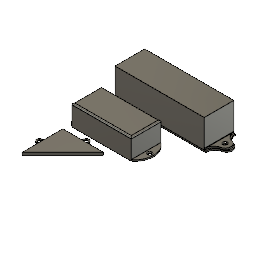
Glow_casings v2 (Autodesk Fusion 360 design; units mm, degrees)
Autodesk Fusion 360 part; units mm, degrees
sketch "Electronic case cap - sketch" plane through (0, 0, 0) normal (0, 1, 0) x (1, 0, 0)
  line L0 (0, 0) -> (137, 0)
  line L1 (0, 0) -> (0, -137)
  line L2 (0, -137) -> (137, 0)
  line L3 (68.5, 0) -> (58.5, 0)
  line L4 (58.5, 0) -> (58.5, 20)
  line L5 (58.5, 20) -> (68.5, 20)
  line L6 (68.5, 20) -> (68.5, 0)
  line L7 (68.5, 0) -> (78.5, 0)
  line L8 (78.5, 0) -> (78.5, 20)
  line L9 (78.5, 20) -> (68.5, 20)
  line L10 (68.5, 20) -> (68.5, 0)
  line L11 (0, -68.5) -> (-20, -68.5)
  line L12 (-20, -68.5) -> (-20, -78.5)
  line L13 (-20, -78.5) -> (0, -78.5)
  line L14 (0, -78.5) -> (0, -68.5)
  line L15 (0, -68.5) -> (-20, -68.5)
  line L16 (-20, -68.5) -> (-20, -58.5)
  line L17 (-20, -58.5) -> (0, -58.5)
  line L18 (0, -58.5) -> (0, -68.5)
  circle A0 centre (68.5, 10) radius 10
  circle A1 centre (68.5, 10) radius 5
  circle A2 centre (-10, -68.5) radius 10
  circle A3 centre (-10, -68.5) radius 5
  dimension "d1" = 137
  dimension "d2" = 137
  dimension "d3" = 10
  dimension "d4" = 20
  dimension "d5" = 20
  dimension "d6" = 10
  dimension "d7" = 20
  dimension "d8" = 10
  dimension "d9" = 10
  dimension "d10" = 20
  dimension "d11" = 10
  dimension "d12" = 10
  constraint coincident L0.start L1.start
  constraint horizontal L0
  constraint perpendicular L0 L1
  constraint horizontal L3
  constraint vertical L4
  constraint horizontal L5
  constraint vertical L6
  constraint midpoint L0 L3.start
  constraint horizontal L7
  constraint vertical L8
  constraint horizontal L9
  constraint vertical L10
  constraint horizontal L11
  constraint vertical L12
  constraint horizontal L13
  constraint vertical L14
  constraint midpoint L1 L11.start
  constraint horizontal L15
  constraint vertical L16
  constraint horizontal L17
  constraint vertical L18
  constraint midpoint L10 A0.centre
  constraint tangent L8 A0
  constraint concentric A0 A1
  constraint midpoint L11 A2.centre
  constraint tangent L17 A2
  constraint concentric A2 A3
  measures "d1" distance of L0.start L0.end
  measures "d2" distance of L0.start L1.end
  measures "d3" distance of L3.start L3.end
  measures "d4" distance of L3.start L5.end
  measures "d5" distance of L3.start L5.end
  measures "d6" distance of L3.start L7.end
  measures "d7" distance of L11.start L11.end
  measures "d8" distance of L11.start L13.end
  measures "d9" distance of L11.start L17.end
  measures "d10" distance of L11.start L11.end
  measures "d11" diameter of A1
  measures "d12" diameter of A3
extrude "Extrude1" add sketch "Electronic case cap - sketch" along normal blind 4 contours L0 L1 L2 L3 L7 L14 L18 | L0 L3 L4 A0 | L1 L17 L18 A2 | L0 L7 L8 A0 | L6 L10 A0 A1 | L6 L10 A0 A1 | L11 L15 A2 A3 | L11 L15 A2 A3 | L1 L13 L14 A2 makes body 1
extrude "Extrude2" add sketch "Electronic case cap - sketch" along normal blind 10 contours L0 L1 L2 L3 L7 L14 L18 bodies 1
sketch "motor case - sketch" plane through (0, 0, 0) normal (0, 1, 0) x (1, 0, 0)
  line L0 (0, 0) -> (200, 0)
  line L1 (200, 0) -> (200, 100)
  line L2 (200, 100) -> (0, 100)
  line L3 (0, 100) -> (0, 0)
  line L4 (0, 100) -> (200, 100) construction
  line L5 (200, 100) -> (200, 0) construction
  line L6 (200, 0) -> (0, 0) construction
  line L7 (0, 0) -> (0, 100) construction
  line L8 (0, 100) -> (14.1421, 85.8579) construction
  line L9 (0, 0) -> (14.1421, 14.1421) construction
  line L10 (200, 100) -> (185.8579, 85.8579) construction
  line L11 (200, 0) -> (185.8789, 14.1631) construction
  circle A0 centre (14.1421, 14.1421) radius 5
  circle A1 centre (14.1421, 85.8579) radius 5
  circle A2 centre (185.8579, 85.8579) radius 5
  line L12 (200, 100) -> (200, 50) construction
  line L13 (200, 50) -> (150, 50) construction
  circle A3 centre (150, 50) radius 11.9947
  circle A4 centre (185.8789, 14.1631) radius 5
  line L14 (200, 0) -> (231.4605, 0)
  line L15 (200, 0) -> (225, 0)
  line L16 (225, 0) -> (225, 100)
  line L17 (225, 100) -> (200, 100)
  line L18 (200, 100) -> (200, 0)
  arc A5 (200, 0) -> (225, 50) centre (162.5, 50) ccw
  arc A6 (225, 50) -> (200, 100) centre (162.5, 50) ccw
  line L19 (225, 50) -> (200, 50) construction
  line L20 (212.5, 50) -> (212.5, 30) construction
  line L21 (212.5, 30) -> (212.5, 50) construction
  line L22 (212.5, 50) -> (212.5, 70) construction
  line L23 (0, 0) -> (-25, 0)
  line L24 (-25, 0) -> (-25, 100)
  line L25 (-25, 100) -> (0, 100)
  line L26 (0, 100) -> (0, 0)
  arc A7 (-25, 50) -> (0, 0) centre (37.5, 50) ccw
  arc A8 (0, 100) -> (-25, 50) centre (37.5, 50) ccw
  line L27 (-25, 50) -> (0, 50) construction
  line L28 (-12.5, 50) -> (-12.5, 30) construction
  line L29 (-12.5, 50) -> (-12.5, 70) construction
  circle A9 centre (212.5, 50) radius 5
  circle A10 centre (-12.5, 50) radius 5
  dimension "d21" = 200
  dimension "d22" = 100
  dimension "d23" = 200
  dimension "d24" = 100
  dimension "d25" = 20
  dimension "d26" = 20
  dimension "d27" = 20
  dimension "d28" = 20
  dimension "d29" = 10
  dimension "d30" = 10
  dimension "d31" = 10
  dimension "d32" = 50
  dimension "d33" = 50
  dimension "d34" = 10
  dimension "d64" = 100
  dimension "d65" = 25
  dimension "d68" = 100
  dimension "d69" = 25
  dimension "d70" = 20
  dimension "d71" = 20
  dimension "d76" = 10
  dimension "d77" = 10
  constraint horizontal L0
  constraint vertical L1
  constraint horizontal L2
  constraint vertical L3
  constraint coincident L0.start L3.end
  constraint horizontal L4
  constraint vertical L5
  constraint horizontal L6
  constraint vertical L7
  constraint coincident L9.end A0.centre
  constraint coincident L8.end A1.centre
  constraint coincident L10.end A2.centre
  constraint vertical L12
  constraint perpendicular L5 L13
  constraint coincident L13.end A3.centre
  constraint coincident L11.end A4.centre
  constraint horizontal L14
  constraint horizontal L15
  constraint vertical L16
  constraint horizontal L17
  constraint vertical L18
  constraint tangent L16 A5
  constraint midpoint L16 A5.end
  constraint tangent L16 A6
  constraint midpoint L19 L20.start
  constraint perpendicular L19 L20
  constraint perpendicular L19 L22
  constraint horizontal L23
  constraint vertical L24
  constraint horizontal L25
  constraint vertical L26
  constraint tangent L24 A7
  constraint tangent L24 A8
  constraint midpoint L7 L27.end
  constraint perpendicular L7 L27
  constraint midpoint L27 L28.start
  constraint perpendicular L27 L28
  constraint perpendicular L27 L29
  constraint coincident L20.start L21.end
  constraint coincident L28.start L29.start
  measures "d21" distance of L0.start L0.end
  measures "d22" distance of L0.start L2.end
  measures "d23" distance of L2.end L1.end
  measures "d24" distance of L2.end L0.start
  measures "d25" distance of L2.end L8.end
  measures "d26" distance of L0.start L9.end
  measures "d27" distance of L1.end L10.end
  measures "d28" distance of L0.end L11.end
  measures "d29" diameter of A0
  measures "d30" diameter of A1
  measures "d31" diameter of A2
  measures "d32" distance of L1.end L12.end
  measures "d33" distance of L12.end L13.end
  measures "d34" diameter of A4
  measures "d64" distance of L0.end L1.end
  measures "d65" distance of L0.end L15.end
  measures "d68" distance of L0.start L2.end
  measures "d69" distance of L0.start L23.end
  measures "d70" distance of L28.start L28.end
  measures "d71" distance of L28.start L29.end
  measures "d76" diameter of A9
  measures "d77" diameter of A10
extrude "Extrude10" add sketch "motor case - sketch" along normal blind 5 separate body contours L3 L26 A7 A8 | L1 L18 A5 A6 | A9 | A10 makes body 2 at (-8.0325, 5, -61.922) makes body 3 at (216.1385, 0, -63.7273)
extrude "Extrude3" add sketch "motor case - sketch" along normal blind 5 separate body contours L0 L1 L2 L3 L18 L26 makes body 4
move_body "Move1" bodies 1 to x (1, 0, 0) y (0, 1, 0) z (0, 0, 1) at (0, 0, 30)
extrude "Extrude4" add sketch "motor case - sketch" along normal blind 70 separate body contours L0 L1 L2 L3 L18 L26 | A0 | A1 | A2 | A3 | A4 makes body 5
shell "Shell1" thickness 5 removed faces 1 at (66.6667, 0, -66.6667) on bodies 5
fillet "Fillet1" radius 5 4 edges at (0, 70, -50) (100, 70, -100) (100, 70, 0) (200, 70, -50) on bodies 5
extrude "Extrude5" cut 1 faces at (133.3333, 1.6667, -100) along direction (0, 0, 1) blind 5.5 on bodies 4 bodies 4
move_face "OffsetFaces1" offset -5.5 1 faces at (200, 1.6667, -31.5) on bodies 4
extrude "Extrude6" cut 1 faces at (64.8333, 1.6667, 0) along direction (0, 0, -1) blind 5.5 on bodies 4 bodies 4
extrude "Extrude7" cut 1 faces at (0, 1.6667, -64.8333) along direction (1, 0, 0) blind 5.5 on bodies 4 bodies 4
sketch "motor case hole - sketch" plane through (0, 0, 0) normal (-1, 0, 0) x (0, 0, 1)
  line L0 (-100, 65) -> (-100, 0)
  line L1 (-100, 0) -> (0, 0)
  line L2 (0, 0) -> (0, 65)
  line L3 (0, 65) -> (-100, 65)
  line L4 (-50, 0) -> (-50, 5)
  circle A0 centre (-50, 15) radius 10
  dimension "d54" = 5
  dimension "d56" = 20
  constraint midpoint L1 L4.start
  constraint perpendicular L1 L4
  constraint coincident L4.end A0
  measures "d54" distance of L4.start L4.end
  measures "d56" diameter of A0
extrude "Extrude9" cut sketch "motor case hole - sketch" against normal blind 10 contours A0 bodies 5
sketch "POWERSUPLY - sketch" plane through (0, 0, 0) normal (0, 1, 0) x (1, 0, 0)
  line L0 (0, 0) -> (300, 0)
  line L1 (300, 0) -> (300, 100)
  line L2 (300, 100) -> (0, 100)
  line L3 (0, 100) -> (0, 0)
  line L4 (340, 70) -> (340, 30)
  line L5 (340, 30) -> (260, 70) construction
  line L6 (260, 30) -> (340, 70) construction
  line L7 (-40, 70) -> (-40, 30)
  line L8 (-40, 30) -> (40, 70) construction
  line L9 (40, 30) -> (-40, 70) construction
  circle A0 centre (-20, 50) radius 20
  circle A1 centre (-20, 50) radius 5
  circle A2 centre (320, 50) radius 20
  circle A3 centre (320, 50) radius 5
  arc A4 (300, 100) -> (320, 70) centre (332.5, 100) ccw
  arc A5 (320, 30) -> (300, 0) centre (332.5, 0) ccw
  arc A6 (-20, 70) -> (0, 100) centre (-32.5, 100) ccw
  arc A7 (0, 0) -> (-20, 30) centre (-32.5, 0) ccw
  line L10 (300, 100) -> (300, 95) construction
  line L11 (0, 0) -> (3.6801, 3.3848) construction
  line L12 (300, 100) -> (296.4645, 96.4645) construction
  line L13 (300, 100) -> (305, 100) construction
  line L14 (296.4645, 96.4645) -> (3.6801, 96.4645)
  line L15 (3.6801, 96.4645) -> (3.6801, 3.3848)
  line L16 (3.6801, 3.3848) -> (296.4645, 3.3848)
  line L17 (296.4645, 3.3848) -> (296.4645, 96.4645)
  line L18 (3.6801, 96.4645) -> (7.2156, 92.9289) construction
  line L19 (3.6801, 96.4645) -> (8.6801, 96.4645) construction
  line L20 (296.4645, 3.3848) -> (292.9289, 6.9203) construction
  line L21 (296.4645, 3.3848) -> (301.4645, 3.3848) construction
  line L22 (292.9289, 6.9203) -> (7.2156, 6.9203)
  line L23 (7.2156, 6.9203) -> (7.2156, 92.9289)
  line L24 (7.2156, 92.9289) -> (292.9289, 92.9289)
  line L25 (292.9289, 92.9289) -> (292.9289, 6.9203)
  point P0 (300, 50)
  point P1 (0, 50)
  dimension "d62" = 300
  dimension "d63" = 100
  dimension "d82" = 10
  dimension "d83" = 10
  dimension "d86" = 5
  dimension "d87" = 5
  dimension "d88" = 135
  dimension "d89" = 5
  dimension "d90" = 5
  dimension "d91" = 45
  dimension "d92" = 135
  dimension "d93" = 5
  constraint horizontal L0
  constraint vertical L1
  constraint horizontal L2
  constraint vertical L3
  constraint coincident L0.start L3.end
  constraint coincident L5 P0
  constraint coincident L6 P0
  constraint midpoint L1 P0
  constraint coincident L8 P1
  constraint coincident L9 P1
  constraint midpoint L3 P1
  constraint coincident P1 A0
  constraint concentric A0 A1
  constraint coincident P0 A2
  constraint tangent L1 A2
  constraint concentric A2 A3
  constraint tangent L1 A4
  constraint coincident A2 A4.end
  constraint tangent L1 A5
  constraint coincident A2 A5.start
  constraint tangent L3 A6
  constraint coincident A0 A6.start
  constraint tangent L3 A7
  constraint coincident A0 A7.end
  constraint perpendicular L2 L10
  constraint horizontal L13
  constraint horizontal L14
  constraint vertical L15
  constraint horizontal L16
  constraint vertical L17
  constraint horizontal L19
  constraint horizontal L21
  constraint horizontal L22
  constraint vertical L23
  constraint horizontal L24
  constraint vertical L25
  measures "d62" distance of L0.start L0.end
  measures "d63" distance of L0.start L2.end
  measures "d82" diameter of A1
  measures "d83" diameter of A3
  measures "d86" distance of L1.end L10.end
  measures "d87" distance of L0.start L11.end
  measures "d88" angle of L12 L13
  measures "d89" distance of L1.end L12.end
  measures "d90" distance of L14.end L18.end
  measures "d91" angle of L18 L19
  measures "d92" angle of L20 L21
  measures "d93" distance of L16.end L20.end
extrude "Extrude12" add sketch "POWERSUPLY - sketch" along normal blind 5 separate body contours L0 L1 L2 L3 | L3 A0 A7 | L1 A2 A5 | L3 A0 A6 | A0 | L1 A2 A4 | A2 | L14 L15 L16 L17 | L22 L23 L24 L25 makes body 6
combine "Combine2" operation add target body 5 tool bodies 3 2
extrude "Extrude11" cut sketch "motor case - sketch" along normal blind 6 contours A9 | A10 bodies 5
chamfer "Chamfer1" distance 2.5 angle 45 2 edges at (-17.1616, 5, -51.8081) (207.8384, 5, -51.8081) on bodies 5
chamfer "Chamfer2" distance 2.5 angle 45 2 edges at (-14.6616, 0, 96.6919) (63.8384, 0, 18.1919) on bodies 1
extrude "Extrude13" add sketch "POWERSUPLY - sketch" along normal blind 10 contours L14 L15 L16 L17 bodies 6
extrude "Extrude14" add sketch "POWERSUPLY - sketch" along normal blind 100 separate body contours L0 L1 L2 L3 | L14 L15 L16 L17 | L22 L23 L24 L25 makes body 7
copy_body "CopyPasteBodies1" bodies 6 makes body 8
shell "Shell2" thickness 5 removed faces 1 at (200, 0, -66.6667) on bodies 7
combine "Combine3" operation cut target body 7 tool bodies 8
extrude "Extrude15" add sketch "POWERSUPLY - sketch" along normal blind 10 contours L3 A0 A7 | L1 A2 A5 | L3 A0 A6 | A0 | L1 A2 A4 | A2 bodies 7
copy_body "CopyPasteBodies2" bodies 6 makes body 9
combine "Combine4" operation cut target body 7 tool bodies 9
sketch "powerSuply case hole - sketch" plane through (300, 0, 0) normal (1, 0, 0) x (0, 0, -1)
  line L0 (0, 10) -> (100, 10)
  line L1 (100, 10) -> (100, 100)
  line L2 (100, 100) -> (0, 100)
  line L3 (0, 100) -> (0, 10)
  line L4 (0, 10) -> (100, 10)
  line L5 (100, 10) -> (100, 100)
  line L6 (100, 100) -> (0, 100)
  line L7 (0, 100) -> (0, 10)
  line L8 (0, 10) -> (7.0711, 17.0711) construction
  circle A0 centre (10.6066, 20.6066) radius 5 construction
  circle A1 centre (10.6066, 20.6066) radius 5
  dimension "d101" = 90
  dimension "d102" = 100
  dimension "d103" = 10
  dimension "d104" = 10
  constraint horizontal L4
  constraint vertical L5
  constraint horizontal L6
  constraint vertical L7
  constraint coincident L0.start L3.end
  constraint coincident L8.end A0
  constraint concentric A0 A1
  measures "d101" distance of L0.start L2.end
  measures "d102" distance of L0.start L0.end
  measures "d103" distance of L0.start L8.end
  measures "d104" diameter of A0
extrude "Extrude16" cut sketch "powerSuply case hole - sketch" against normal blind 15 contours A1 bodies 7
chamfer "Chamfer3" distance 2.5 angle 45 2 edges at (315.3384, 10, -51.8081) (-24.6616, 10, -51.8081) on bodies 7
move_body "Move3" bodies 6 7 to x (1, 0, 0) y (0, 1, 0) z (0, 0, 1) at (0, 0, -150)
move_body "Move4" bodies 7 to x (-1, 0, 0) y (0, 1, 0) z (0, 0, -1) at (-80, 0, -500)
move_body "Move5" bodies 7 to x (1, 0, 0) y (0, 1, 0) z (0, 0, 1) at (375, 0, 100)
equation "motor_case_width = 100 mm"
equation "motor_case_length = 200 mm"
equation "motor_case_height = 70 mm"
equation "d21 = motor_case_length"
equation "d22 = motor_case_width"
equation "d23 = motor_case_length"
equation "d32 = motor_case_width / 2"
equation "d37 = motor_case_height"
equation "motor_tube_size = 20 mm"
equation "d56 = motor_tube_size"
equation "powerSuply_width = 100 mm"
equation "powerSuply_length = 300 mm"
equation "powerSuply_height = 100 mm"
equation "d62 = powerSuply_length"
equation "d63 = powerSuply_width"
equation "d64 = motor_case_width"
equation "d68 = motor_case_width"
equation "d96 = powerSuply_height"
equation "d101 = powerSuply_height - 10 mm"
equation "d102 = powerSuply_width"
named bodies: "Electronic case cap", "motor_case_floor", "motor_case_cap", "powerSuply_floor", "powerSuply_cap", "powerSuply_floor (1)"
